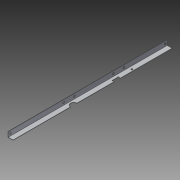
# Autodesk Inventor part: Shooter Side Support Bar - L
Saved by Autodesk Inventor 2014 SP1 (Build 180222100, 222)
## iProperties
Created: 2013-12-13
Part Number: Shooter Side Support Bar - L
Material: Aluminum 6061
Document SubType Name: Modeling
Designer: Moses
Mass: 31.8794 g
Surface Area: 306.093 cm^2
Volume: 11.7636 cm^3
Density: 2.71 g/cm^3
Appearance: Aluminum - Flat
Author: Moses
Autodesk Inventor part; units mm, degrees
ref_plane "YZ Plane" through (0, 0, 0) normal (1, 0, 0) x (0, 1, 0)
ref_plane "XZ Plane" through (0, 0, 0) normal (0, 1, 0) x (-1, 0, 0)
ref_plane "XY Plane" through (0, 0, 0) normal (0, 0, 1) x (1, 0, 0)
sketch "Sketch1" plane through (0, 0, 0) normal (0, 0, 1) x (1, 0, 0)
  line L0 (0, 0) -> (0, 15.875)
  line L1 (0, 15.875) -> (0.7937, 15.875)
  line L2 (0.7937, 15.875) -> (0.7938, 0.7937)
  line L3 (0.7938, 0.7937) -> (15.875, 0.7937)
  line L4 (15.875, 0.7937) -> (15.875, 0)
  line L5 (15.875, 0) -> (0, 0)
  dimension "d0" = 15.875
  dimension "d1" = 0.7937
  constraints: 12 end point, 3 horizontal, 3 vertical, 2 perpendicular
  measures "d0" distance of L0.start L0.end
  measures "d1" distance of L0.end L1.end
extrude "Extrusion1" add sketch "Sketch1" along normal blind 495.3
sketch "Sketch2" plane through (0, 0, 0) normal (0, -1, 0) x (1, 0, 0)
  line L0 (15.875, 0) -> (15.875, 495.3) projected
  line L1 (14.2875, 178.5938) -> (14.2875, 162.7188) construction
  line L2 (14.2875, 162.7188) -> (15.0813, 162.7188) construction
  line L3 (15.0813, 162.7188) -> (15.0813, 177.8) construction
  line L4 (15.0813, 177.8) -> (30.1625, 177.8) construction
  line L5 (30.1625, 177.8) -> (30.1625, 178.5938) construction
  line L6 (30.1625, 178.5938) -> (14.2875, 178.5938) construction
  line L7 (15.875, 161.1313) -> (9.525, 161.1313)
  line L8 (9.525, 161.1313) -> (9.525, 180.1813)
  line L9 (9.525, 180.1813) -> (15.875, 180.1813)
  line L10 (14.2875, 170.6563) -> (15.875, 170.6563) construction
  circle A0 centre (10.3187, 179.3875) radius 1.5875
  circle A1 centre (10.3187, 161.925) radius 1.5875
  circle A2 centre (10.3187, 119.38) radius 1.905 projected
  circle A3 centre (16.7716, 306.2288) radius 8.255 projected
  arc A4 (22.0116, 315.7538) -> (11.5316, 315.7538) centre (16.7716, 306.2288) ccw construction
  line L11 (11.5316, 315.7538) -> (22.0116, 315.7538) projected
  arc A5 (11.5316, 296.7038) -> (22.0116, 296.7038) centre (16.7716, 306.2288) ccw construction
  line L12 (22.0116, 296.7038) -> (11.5316, 296.7038) projected
  arc A6 (22.0116, 296.7038) -> (22.0116, 315.7538) centre (16.7716, 306.2288) ccw
  arc A7 (11.5316, 315.7538) -> (11.5316, 296.7038) centre (16.7716, 306.2288) ccw
  point P0 (9.525, 170.6563)
  dimension "d4" = 6.35
  dimension "d5" = 19.05
  dimension "d8" = 3.175
  dimension "d9" = 0.7937
  dimension "d10" = 0.7937
  dimension "d11" = 0.7937
  dimension "d12" = 0.7937
  constraints: 8 end point, 4 centre point, 4 point on circle, 4 point on line, 3 horizontal, 2 coincident, 2 midpoint, 1 equal radius, 1 vertical
  measures "d4" distance of L7.start L7.end
  measures "d5" distance of L7.end L8.end
  measures "d8" diameter of A0
  measures "d9" distance from line of L9 A0.centre
  measures "d10" distance from line of L8 A0.centre
  measures "d11" distance from line of L7 A1.centre
  measures "d12" distance from line of A1.centre L8
extrude "Extrusion2" cut sketch "Sketch2" against normal through all
sketch "Sketch3" plane through (0, 0, 0) normal (-1, 0, 0) x (0, 0, 1)
  line L0 (219.2782, 408.7812) -> (219.2782, 103.9812) construction
  arc A0 (212.5218, 103.9812) -> (219.2782, 103.9812) centre (215.9, 103.9812) ccw construction
  line L1 (212.5218, 103.9812) -> (212.5218, 408.7812) construction
  arc A1 (219.2782, 408.7812) -> (212.5218, 408.7812) centre (215.9, 408.7812) ccw construction
  circle A2 centre (215.9, 472.2812) radius 3.3782 construction
  circle A3 centre (215.9, 440.5312) radius 3.3782 construction
  line L2 (228.6, 484.9812) -> (330.2, 484.9812) construction
  line L3 (330.2, 484.9812) -> (330.2, 15.0812) construction
  line L4 (330.2, 15.0812) -> (228.6, 15.0812) construction
  line L5 (228.6, 484.9812) -> (228.6, 15.0812) construction
  line L6 (346.2782, 408.7812) -> (346.2782, 103.9812) construction
  arc A4 (339.5218, 103.9812) -> (346.2782, 103.9812) centre (342.9, 103.9812) ccw construction
  line L7 (339.5218, 103.9812) -> (339.5218, 408.7812) construction
  arc A5 (346.2782, 408.7812) -> (339.5218, 408.7812) centre (342.9, 408.7812) ccw construction
  line L8 (495.3, 2.3812) -> (495.3, 497.6812) construction
  line L9 (495.3, 497.6812) -> (0, 497.6812) construction
  line L10 (0, 497.6812) -> (0, 2.3812) construction
  line L11 (0, 2.3812) -> (495.3, 2.3812) construction
  circle A6 centre (488.95, 8.7313) radius 3.3782 projected
  circle A7 centre (488.95, 18.5802) radius 3.3782 construction
  circle A8 centre (488.95, 28.4292) radius 3.3782 construction
  circle A9 centre (488.95, 38.2782) radius 3.3782 construction
  circle A10 centre (488.95, 48.1272) radius 3.3782 construction
  circle A11 centre (488.95, 57.9761) radius 3.3782 construction
  circle A12 centre (488.95, 67.8251) radius 3.3782 construction
  circle A13 centre (488.95, 77.6741) radius 3.3782 construction
  circle A14 centre (488.95, 87.5231) radius 3.3782 construction
  circle A15 centre (488.95, 117.07) radius 3.3782 construction
  circle A16 centre (488.95, 126.919) radius 3.3782 construction
  circle A17 centre (488.95, 136.768) radius 3.3782 construction
  circle A18 centre (488.95, 146.617) radius 3.3782 construction
  circle A19 centre (488.95, 156.4659) radius 3.3782 construction
  circle A20 centre (488.95, 166.3149) radius 3.3782 construction
  circle A21 centre (488.95, 176.1639) radius 3.3782 construction
  circle A22 centre (488.95, 186.0129) radius 3.3782 construction
  circle A23 centre (488.95, 195.8619) radius 3.3782 construction
  circle A24 centre (488.95, 205.7108) radius 3.3782 construction
  circle A25 centre (488.95, 215.5598) radius 3.3782 construction
  circle A26 centre (488.95, 225.4088) radius 3.3782 construction
  circle A27 centre (488.95, 235.2578) radius 3.3782 construction
  circle A28 centre (488.95, 245.1068) radius 3.3782 construction
  circle A29 centre (488.95, 254.9557) radius 3.3782 construction
  circle A30 centre (488.95, 264.8047) radius 3.3782 construction
  circle A31 centre (488.95, 274.6537) radius 3.3782 construction
  circle A32 centre (488.95, 284.5027) radius 3.3782 construction
  circle A33 centre (488.95, 294.3517) radius 3.3782 construction
  circle A34 centre (488.95, 304.2006) radius 3.3782 construction
  circle A35 centre (488.95, 314.0496) radius 3.3782 construction
  circle A36 centre (488.95, 323.8986) radius 3.3782 construction
  circle A37 centre (488.95, 333.7476) radius 3.3782 construction
  circle A38 centre (488.95, 343.5966) radius 3.3782 construction
  circle A39 centre (488.95, 353.4455) radius 3.3782 construction
  circle A40 centre (488.95, 363.2945) radius 3.3782 construction
  circle A41 centre (488.95, 373.1435) radius 3.3782 construction
  circle A42 centre (488.95, 382.9925) radius 3.3782 construction
  circle A43 centre (488.95, 392.8415) radius 3.3782 construction
  circle A44 centre (488.95, 402.6904) radius 3.3782 construction
  circle A45 centre (488.95, 412.5394) radius 3.3782 construction
  circle A46 centre (488.95, 422.3884) radius 3.3782 construction
  circle A47 centre (488.95, 432.2374) radius 3.3782 construction
  circle A48 centre (488.95, 442.0864) radius 3.3782 construction
  circle A49 centre (488.95, 451.9353) radius 3.3782 construction
  circle A50 centre (488.95, 461.7843) radius 3.3782 construction
  circle A51 centre (488.95, 471.6333) radius 3.3782 construction
  circle A52 centre (488.95, 481.4823) radius 3.3782 construction
  circle A53 centre (488.95, 491.3312) radius 3.3782 construction
  circle A54 centre (6.35, 8.7312) radius 3.3782 projected
  circle A55 centre (6.35, 18.5802) radius 3.3782 construction
  circle A56 centre (6.35, 28.4292) radius 3.3782 construction
  circle A57 centre (6.35, 38.2782) radius 3.3782 construction
  circle A58 centre (6.35, 48.1272) radius 3.3782 construction
  circle A59 centre (6.35, 57.9761) radius 3.3782 construction
  circle A60 centre (6.35, 67.8251) radius 3.3782 construction
  circle A61 centre (6.35, 77.6741) radius 3.3782 construction
  circle A62 centre (6.35, 87.5231) radius 3.3782 construction
  circle A63 centre (6.35, 97.3721) radius 3.3782 construction
  circle A64 centre (6.35, 107.221) radius 3.3782 construction
  circle A65 centre (6.35, 117.07) radius 3.3782 construction
  circle A66 centre (6.35, 126.919) radius 3.3782 construction
  circle A67 centre (6.35, 136.768) radius 3.3782 construction
  circle A68 centre (6.35, 146.617) radius 3.3782 construction
  circle A69 centre (6.35, 156.4659) radius 3.3782 construction
  circle A70 centre (6.35, 166.3149) radius 3.3782 construction
  circle A71 centre (6.35, 176.1639) radius 3.3782 construction
  circle A72 centre (6.35, 186.0129) radius 3.3782 construction
  circle A73 centre (6.35, 195.8619) radius 3.3782 construction
  circle A74 centre (6.35, 205.7108) radius 3.3782 construction
  circle A75 centre (6.35, 215.5598) radius 3.3782 construction
  circle A76 centre (6.35, 225.4088) radius 3.3782 construction
  circle A77 centre (6.35, 235.2578) radius 3.3782 construction
  circle A78 centre (6.35, 245.1068) radius 3.3782 construction
  circle A79 centre (6.35, 254.9557) radius 3.3782 construction
  circle A80 centre (6.35, 264.8047) radius 3.3782 construction
  circle A81 centre (6.35, 274.6537) radius 3.3782 construction
  circle A82 centre (6.35, 284.5027) radius 3.3782 construction
  circle A83 centre (6.35, 294.3517) radius 3.3782 construction
  circle A84 centre (6.35, 304.2006) radius 3.3782 construction
  circle A85 centre (6.35, 314.0496) radius 3.3782 construction
  circle A86 centre (6.35, 323.8986) radius 3.3782 construction
  circle A87 centre (6.35, 333.7476) radius 3.3782 construction
  circle A88 centre (6.35, 343.5966) radius 3.3782 construction
  circle A89 centre (6.35, 353.4455) radius 3.3782 construction
  circle A90 centre (6.35, 363.2945) radius 3.3782 construction
  circle A91 centre (6.35, 373.1435) radius 3.3782 construction
  circle A92 centre (6.35, 382.9925) radius 3.3782 construction
  circle A93 centre (6.35, 392.8415) radius 3.3782 construction
  circle A94 centre (6.35, 402.6904) radius 3.3782 construction
  circle A95 centre (6.35, 412.5394) radius 3.3782 construction
  circle A96 centre (6.35, 422.3884) radius 3.3782 construction
  circle A97 centre (6.35, 432.2374) radius 3.3782 construction
  circle A98 centre (6.35, 442.0864) radius 3.3782 construction
  circle A99 centre (6.35, 451.9353) radius 3.3782 construction
  circle A100 centre (6.35, 461.7843) radius 3.3782 construction
  circle A101 centre (6.35, 471.6333) radius 3.3782 construction
  circle A102 centre (6.35, 481.4823) radius 3.3782 construction
  circle A103 centre (6.35, 491.3312) radius 3.3782 construction
  circle A104 centre (477.8829, 8.7313) radius 3.3782 construction
  circle A105 centre (477.8829, 491.3312) radius 3.3782 construction
  circle A106 centre (466.8157, 8.7313) radius 3.3782 construction
  circle A107 centre (466.8157, 491.3312) radius 3.3782 construction
  circle A108 centre (455.7486, 8.7313) radius 3.3782 construction
  circle A109 centre (455.7486, 491.3312) radius 3.3782 construction
  circle A110 centre (444.6814, 8.7313) radius 3.3782 construction
  circle A111 centre (444.6814, 491.3312) radius 3.3782 construction
  circle A112 centre (433.6143, 8.7313) radius 3.3782 construction
  circle A113 centre (433.6143, 491.3312) radius 3.3782 construction
  circle A114 centre (422.5471, 8.7313) radius 3.3782 construction
  circle A115 centre (422.5471, 491.3312) radius 3.3782 construction
  circle A116 centre (411.48, 8.7313) radius 3.3782 construction
  circle A117 centre (411.48, 491.3312) radius 3.3782 construction
  circle A118 centre (400.4129, 8.7313) radius 3.3782 construction
  circle A119 centre (400.4129, 491.3312) radius 3.3782 construction
  circle A120 centre (389.3457, 8.7313) radius 3.3782 construction
  circle A121 centre (389.3457, 491.3312) radius 3.3782 construction
  circle A122 centre (378.2786, 8.7313) radius 3.3782 construction
  circle A123 centre (378.2786, 491.3312) radius 3.3782 construction
  circle A124 centre (367.2114, 8.7313) radius 3.3782 construction
  circle A125 centre (367.2114, 491.3312) radius 3.3782 construction
  circle A126 centre (356.1443, 8.7313) radius 3.3782 construction
  circle A127 centre (356.1443, 491.3312) radius 3.3782 construction
  circle A128 centre (345.0771, 8.7313) radius 3.3782 construction
  circle A129 centre (345.0771, 491.3312) radius 3.3782 construction
  circle A130 centre (334.01, 8.7313) radius 3.3782 construction
  circle A131 centre (334.01, 491.3312) radius 3.3782 construction
  circle A132 centre (322.9429, 8.7313) radius 3.3782 projected
  circle A133 centre (322.9429, 491.3312) radius 3.3782 construction
  circle A134 centre (311.8757, 8.7313) radius 3.3782 construction
  circle A135 centre (311.8757, 491.3312) radius 3.3782 construction
  circle A136 centre (300.8086, 8.7313) radius 3.3782 construction
  circle A137 centre (300.8086, 491.3312) radius 3.3782 construction
  circle A138 centre (289.7414, 8.7313) radius 3.3782 projected
  circle A139 centre (289.7414, 491.3312) radius 3.3782 construction
  circle A140 centre (278.6743, 8.7313) radius 3.3782 construction
  circle A141 centre (278.6743, 491.3312) radius 3.3782 construction
  circle A142 centre (267.6071, 8.7313) radius 3.3782 construction
  circle A143 centre (267.6071, 491.3312) radius 3.3782 construction
  circle A144 centre (256.54, 8.7313) radius 3.3782 construction
  circle A145 centre (256.54, 491.3312) radius 3.3782 construction
  circle A146 centre (245.4729, 8.7313) radius 3.3782 construction
  circle A147 centre (245.4729, 491.3312) radius 3.3782 construction
  circle A148 centre (234.4057, 8.7313) radius 3.3782 construction
  circle A149 centre (234.4057, 491.3312) radius 3.3782 construction
  circle A150 centre (223.3386, 8.7313) radius 3.3782 construction
  circle A151 centre (223.3386, 491.3312) radius 3.3782 construction
  circle A152 centre (212.2714, 8.7313) radius 3.3782 construction
  circle A153 centre (212.2714, 491.3312) radius 3.3782 construction
  circle A154 centre (201.2043, 8.7313) radius 3.3782 construction
  circle A155 centre (201.2043, 491.3312) radius 3.3782 construction
  circle A156 centre (190.1371, 8.7313) radius 3.3782 construction
  circle A157 centre (190.1371, 491.3312) radius 3.3782 construction
  circle A158 centre (179.07, 8.7313) radius 3.3782 construction
  circle A159 centre (179.07, 491.3312) radius 3.3782 construction
  circle A160 centre (168.0029, 8.7313) radius 3.3782 projected
  circle A161 centre (168.0029, 491.3312) radius 3.3782 construction
  circle A162 centre (156.9357, 8.7313) radius 3.3782 construction
  circle A163 centre (156.9357, 491.3312) radius 3.3782 construction
  circle A164 centre (145.8686, 8.7313) radius 3.3782 construction
  circle A165 centre (145.8686, 491.3312) radius 3.3782 construction
  circle A166 centre (134.8014, 8.7313) radius 3.3782 projected
  circle A167 centre (134.8014, 491.3312) radius 3.3782 construction
  circle A168 centre (123.7343, 8.7313) radius 3.3782 construction
  circle A169 centre (123.7343, 491.3312) radius 3.3782 construction
  circle A170 centre (112.6671, 8.7313) radius 3.3782 construction
  circle A171 centre (112.6671, 491.3312) radius 3.3782 construction
  circle A172 centre (18.2563, 8.7312) radius 3.3782 construction
  circle A173 centre (18.2563, 491.3312) radius 3.3782 construction
  circle A174 centre (30.1625, 8.7312) radius 3.3782 construction
  circle A175 centre (30.1625, 491.3312) radius 3.3782 construction
  circle A176 centre (42.0688, 8.7312) radius 3.3782 construction
  circle A177 centre (42.0688, 491.3312) radius 3.3782 construction
  circle A178 centre (53.975, 8.7312) radius 3.3782 construction
  circle A179 centre (53.975, 491.3312) radius 3.3782 construction
  circle A180 centre (65.8813, 8.7312) radius 3.3782 construction
  circle A181 centre (65.8813, 491.3312) radius 3.3782 construction
  circle A182 centre (77.7875, 8.7312) radius 3.3782 construction
  circle A183 centre (77.7875, 491.3312) radius 3.3782 construction
  circle A184 centre (89.6938, 8.7312) radius 3.3782 construction
  circle A185 centre (89.6938, 491.3312) radius 3.3782 construction
  circle A186 centre (101.6, 8.7312) radius 3.3782 construction
  circle A187 centre (101.6, 491.3312) radius 3.3782 construction
  line L12 (203.2, 15.0812) -> (203.2, 484.9812) construction
  line L13 (203.2, 15.0812) -> (12.7, 15.0812) construction
  line L14 (12.7, 15.0812) -> (12.7, 484.9812) construction
  line L15 (12.7, 484.9812) -> (203.2, 484.9812) construction
  line L16 (355.6, 484.9812) -> (482.6, 484.9812) construction
  line L17 (482.6, 484.9812) -> (482.6, 15.0812) construction
  line L18 (482.6, 15.0812) -> (355.6, 15.0812) construction
  line L19 (355.6, 15.0812) -> (355.6, 484.9812) construction
  arc A188 (487.5398, 100.4418) -> (490.3602, 100.4418) centre (488.95, 97.3721) ccw projected
  arc A189 (492.1297, 106.0802) -> (485.7703, 106.0802) centre (488.95, 107.221) ccw projected
  arc A190 (485.7703, 106.0802) -> (487.5398, 100.4418) centre (488.95, 103.9812) ccw projected
  arc A191 (490.3602, 100.4418) -> (492.1297, 106.0802) centre (488.95, 103.9812) ccw projected
  ellipse E0 centre (342.9016, 472.2812) end of major axis (342.9016, 468.903) minor radius 3.3782 projected
  ellipse E1 centre (342.9016, 440.5312) end of major axis (342.9016, 443.9094) minor radius 3.3782 projected
  constraints: 2 other
extrude "Extrusion3" cut sketch "Sketch3" against normal through all contours A6 | A54 | A132 | A138 | A160 | A166
equation "\"d10\" = d9"
equation "\"d11\" = d10"
equation "\"d12\" = d11"
body "Solid1"
